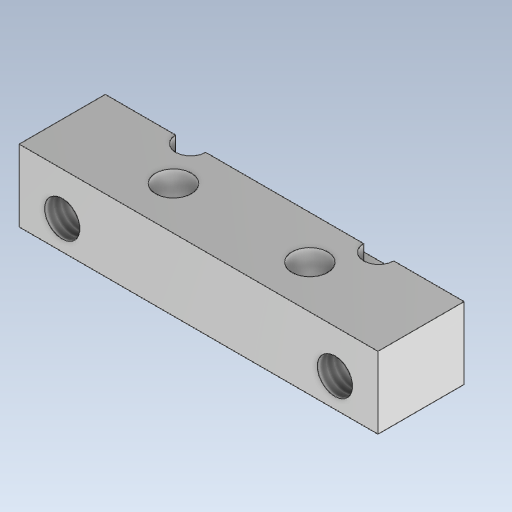
# Autodesk Inventor part: Foot_root_block
Saved by Autodesk Inventor 2020.4 (Build 244396000, 396)
## iProperties
Created: 2022-01-10
Part Number: Foot_root_block
Material: アルミニウム 2014-T4
Document SubType Name: Modeling
Designer: Masato Kubotera
Density: 2.8 g/cm^3
Appearance: 滑らか - 淡い灰色
Description: A2017 T5
Mass: 1.9085 g
Surface Area: 8.0167 cm^2
Volume: 0.681606 cm^3
Author: Masato Kubotera
Autodesk Inventor part; units mm, degrees
ref_plane "YZ Plane" through (0, 0, 0) normal (1, 0, 0) x (0, 1, 0)
ref_plane "XZ Plane" through (0, 0, 0) normal (0, 1, 0) x (-1, 0, 0)
ref_plane "XY Plane" through (0, 0, 0) normal (0, 0, 1) x (1, 0, 0)
sketch "スケッチ1" plane through (0, 0, 0) normal (0, 0, 1) x (1, 0, 0)
  line L0 (0, -5.5) -> (0, 5.5)
  line L1 (0, -5.5) -> (2, -5.5)
  line L2 (2, -7.6) -> (2, -12.5)
  line L3 (2, -12.5) -> (8, -12.5)
  line L4 (8, -12.5) -> (8, 12.5)
  line L5 (0, 0) -> (8, 0) construction
  arc A0 (2, -7.6) -> (2, -5.5) centre (2, -6.55) ccw
  line L6 (2, -9.5) -> (8, -9.5) construction
  line L7 (2, -11) -> (8, -11) construction
  line L8 (2, -8) -> (8, -8) construction
  line L9 (0, 5.5) -> (2, 5.5)
  line L10 (2, 7.6) -> (2, 12.5)
  line L11 (2, 12.5) -> (8, 12.5)
  arc A1 (2, 5.5) -> (2, 7.6) centre (2, 6.55) ccw
  line L12 (2, 9.5) -> (8, 9.5) construction
  line L13 (2, 11) -> (8, 11) construction
  line L14 (2, 8) -> (8, 8) construction
  circle A2 centre (5, -4.75) radius 1.25
  circle A3 centre (5, 4.75) radius 1.25
  line L15 (5, -12.5) -> (5, 12.5) construction
  line L16 (2, 5.5) -> (2, -5.5)
  dimension "d0" = 2
  dimension "d1" = 6
  dimension "d2" = 1.05
  dimension "d3" = 11
  dimension "d4" = 25
  dimension "d5" = 3
  dimension "d6" = 19
  dimension "d7" = 2.5
  dimension "d9" = 9.5
  constraints: 34 end point, 13 symmetric about line, 9 point on line, 4 centre point, 4 midpoint, 4 perpendicular, 4 point on circle, 3 horizontal, 2 vertical, 1 tangent, 2 other
  measures "d0" distance of L1.end L0.start
  measures "d1" distance of L2.end L3.end
  measures "d2" radius of A0
  measures "d3" distance of L0.start L0.end
  measures "d4" distance of L3.end L4.end
  measures "d5" distance of L7.start L8.start
  measures "d6" distance of L12.end L6.end
  measures "d7" diameter of A2
  measures "d9" distance of A3.centre A2.centre
extrude "押し出し1" add sketch "スケッチ1" along normal blind 5 contours L16 A1 L10 L11 L4 L3 L2 A0
extrude "押し出し2" add sketch "スケッチ1" along normal blind 2.5 contours L0 L9 L16 L1
sketch "スケッチ2" plane through (8, -12.5, 0) normal (1, 0, 0) x (0, 0, -1)
  line L0 (0, 12.5) -> (-5, 12.5) construction
  line L1 (-5, 0) -> (-5, 25) projected
  line L2 (0, 0) -> (-5, 0) projected
  line L3 (0, 25) -> (-5, 25) projected
  line L4 (-2, 0) -> (-2, 25) construction
  point P0 (-2, 3)
  point P1 (-2, 22)
  dimension "d13" = 19
  dimension "d23" = 3
  constraints: 4 end point, 3 point on line, 1 midpoint, 1 perpendicular, 1 symmetric about line
  measures "d13" distance of point (-2, 22) point (-2, 3)
  measures "d23" distance of L4.start L1.start
hole "穴1" at (8, -9.5, 2) at (8, 9.5, 2) direction (-1, 0, 0) diameter 2.459 depth 6 tip angle 118 thread size "M3x0.5" class "6H" standard "ISO Metric profile"
equation "\"d13\" = d6"
